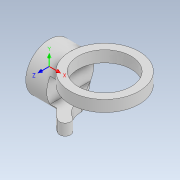
# Autodesk Inventor part: hip_front_left
Saved by Autodesk Inventor 2020 (Build 240168000, 168)
## iProperties
Created: 2021-01-12
Part Number: hip_front_left
Material: Generic
Document SubType Name: Modeling
Designer: DELL
Density: 1 g/cm^3
Appearance: Default
Author: DELL
Autodesk Inventor part; units mm, degrees
ref_plane "YZ Plane" through (0, 0, 0) normal (1, 0, 0) x (0, 1, 0)
ref_plane "XY Plane" through (0, 0, 0) normal (0, 0, 1) x (1, 0, 0)
ref_plane "UCS1: YZ Plane" through (0, 0, 0) normal (1, 0, 0) x (0, 1, 0)
sketch "Sketch1" plane through (0, 0, 0) normal (1, 0, 0) x (0, 1, 0)
  line L0 (0, 0) -> (0, -9.715) construction
  circle A0 centre (0, 0) radius 17.5 construction
  circle A1 centre (0, 0) radius 28
  line L1 (0, 0) -> (0, 11.5) construction
  line L2 (14.5, 23.9531) -> (14.5, -23.9531)
  line L3 (-14.5, 23.9531) -> (-14.5, -23.9531)
  line L4 (0, 28) -> (0, -28) construction
  line L5 (-14.5, 0) -> (-28, 0)
  line L6 (-28, -23.9531) -> (-28, 0)
  arc A2 (-18.6667, -20.87) -> (-14.5, -19.0066) centre (-17, -19.0066) ccw
  line L7 (-28, -23.9531) -> (-14.5, -23.9531)
  dimension "d5" = 56
  dimension "d4" = 35
  dimension "d7" = 29
  dimension "d10" = 5
  constraints: 16 end point, 5 coincident, 3 midpoint, 3 point on line, 3 vertical, 2 centre point, 2 horizontal, 2 point on circle, 1 parallel, 1 tangent, 12 other
  measures "d4" diameter of A0
  measures "d7" distance between parallel lines of L3 L2
  measures "d10" diameter of A2
extrude "Extrusion1" add sketch "Sketch1" along normal blind 25 contours A1 L2 | L2 A1 L3 | L3 L5 A1 | A1 A2 L3 | L5 L3 A2 A1
sketch "Sketch2" plane through (0, 0, 0) normal (0, 1, 0) x (-1, 0, 0)
  line L0 (-107, 0) -> (-25, 0) construction
  circle A0 centre (-66, 0) radius 28
  circle A1 centre (-66, 0) radius 31.5
  circle A2 centre (-66, 0) radius 41 construction
  circle A3 centre (-66, 0) radius 41
  line L1 (-45.5, 35.507) -> (-66, 0) construction
  line L2 (0, -28) -> (0, 28) construction
  line L3 (-66, 41) -> (-66, -41) construction
  circle A4 centre (-48.75, 29.8779) radius 6.5
  circle A5 centre (-31.5, 0) radius 6.5
  line L4 (-25, 28) -> (-25, -28) projected
  point P0 (0, 0)
  point P1 (0, 0)
  point P2 (-45.5, 35.507)
  point P3 (-52, 24.2487)
  point P4 (-38, 0)
  point P5 (-25, 0)
  dimension "d22" = 82
  dimension "d23" = 56
  dimension "d24" = 63
  dimension "d31" = 60
  constraints: 8 end point, 6 centre point, 5 midpoint, 5 point on circle, 5 tangent, 4 coincident, 2 horizontal alignment, 2 point on line, 1 concentric, 1 horizontal, 1 vertical
  measures "d22" diameter of A2
  measures "d23" diameter of A0
  measures "d24" diameter of A1
  measures "d31" angle of L0 L1
ref_plane "Work Plane1" through (0, 14.5, 0) normal (0, 1, 0) x (-1, 0, 0)
ref_plane "Work Plane2" through (0, -14.5, 0) normal (0, 1, 0) x (-1, 0, 0)
extrude "Extrusion2" add sketch "Sketch2" along normal blind 13.5 from surface at 14.5 contours A5 A1 | A1 A4 A3 A5 | A5 A3 A4 A1 | A4 A1 picked at (-31.8776, -2.0283) picked at (-48.6846, 29.9912)
extrude "Extrusion3" add sketch "Sketch2" against normal blind 13.5 from surface at -14.5 contours A0 A4 A1 A5 | A5 A1 | A4 A1 | A5 A1 | A1 A4 A3 A5 | A4 A1 picked at (-40.3852, 15.9153) picked at (-36.5177, 17.9392)
extrude "Extrusion4" add sketch "Sketch1" along normal up to surface from surface at 25 contours A1 L2 | L3 L5 A1 round surface about axis through (66, 0, 0) along (0, 1, 0) radius 41 far side no
sketch "Sketch3" plane through (31.5, -28, 0) normal (0, -1, 0) x (1, 0, 0)
  line L0 (-6.5, 23.9531) -> (-6.5, 0) projected
  line L1 (-6.5, -23.9531) -> (-6.5, 23.9531) projected
  line L2 (-6.5, 0) -> (-6.5, -23.9531)
  line L3 (-6.5, -23.9531) -> (5.6084, -3.2858)
  arc A0 (-6.5, 0) -> (6.5, 0) centre (0, 0) ccw projected
  point P0 (-31.5, 0)
  constraints: 4 end point, 1 point on circle, 1 tangent, 1 vertical
extrude "Extrusion5" add sketch "Sketch3" against normal up to surface (13.5 mm away)
extrude "Extrusion6" cut sketch "Sketch1" along normal through all contours L7 L6 A1
body "Solid1"
